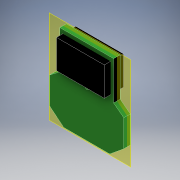
# Autodesk Inventor part: Probe
Saved by Autodesk Inventor 2020 (Build 240168000, 168)
## iProperties
Created: 2020-07-27
Part Number: Probe
Material: 일반
Document SubType Name: Modeling
Designer: Knowblesse
Density: 1 g/cm^3
Appearance: 기본값
Author: Knowblesse
Autodesk Inventor part; units mm, degrees
ref_plane "YZ Plane" through (0, 0, 0) normal (1, 0, 0) x (0, 1, 0)
ref_plane "XZ Plane" through (0, 0, 0) normal (0, 1, 0) x (-1, 0, 0)
ref_plane "XY Plane" through (0, 0, 0) normal (0, 0, 1) x (1, 0, 0)
sketch "스케치1" plane through (0, 0, 0) normal (0, 0, 1) x (1, 0, 0)
  line L0 (-3.5, -3) -> (3.5, -3)
  line L1 (3.5, -3) -> (3.5, 3)
  line L2 (3.5, 3) -> (-3.5, 3)
  line L3 (-3.5, 3) -> (-3.5, -3)
  line L4 (-3.5, -3) -> (3.5, 3) construction
  line L5 (3.5, -3) -> (-3.5, 3) construction
  line L6 (-4.825, -6.5) -> (4.825, -6.5)
  line L7 (4.825, -6.5) -> (4.825, -3)
  line L8 (4.825, -3) -> (-4.825, -3)
  line L9 (-4.825, -3) -> (-4.825, -6.5)
  line L10 (-4.825, -6.5) -> (4.825, -3) construction
  line L11 (4.825, -6.5) -> (-4.825, -3) construction
  line L12 (-4.825, -6.5) -> (-3, -8)
  line L13 (-3, -8) -> (3, -8)
  line L14 (3, -8) -> (4.825, -6.5)
  line L15 (4.825, -3) -> (3.5, -2)
  line L16 (-4.825, -3) -> (-3.5, -2)
  point P0 (0, 0)
  point P1 (0, -4.75)
  point P2 (0, -8)
  point P3 (0, -6.5)
  point P4 (0, 0)
  point P5 (0, -3)
  dimension "d0" = 7
  dimension "d1" = 6
  dimension "d2" = 9.65
  dimension "d3" = 3.5
  dimension "d4" = 1.5
  dimension "d5" = 6
  dimension "d7" = 1
  constraints: 34 end point, 9 midpoint, 4 parallel, 3 horizontal, 3 vertical alignment, 2 perpendicular, 2 point on line, 1 horizontal alignment
  measures "d0" distance of L2.end L1.end
  measures "d1" distance of L1.end L0.end
  measures "d2" distance of L8.end L7.end
  measures "d3" distance of L7.end L6.end
  measures "d4" distance between parallel lines of L6 L13
  measures "d5" distance of L12.end L13.end
  measures "d7" distance from line of L15.end L8
extrude "돌출1" add sketch "스케치1" along normal blind 0.85
ref_plane "작업 평면2" through (0, 0, 0.425) normal (0, 0, 1) x (1, 0, 0)
sketch "스케치4" plane through (0, 0, 0.425) normal (0, 0, 1) x (1, 0, 0)
  line L0 (3.11, 2.5) -> (-3.11, 2.5)
  line L1 (-3.11, 2.5) -> (-3.11, -1.26)
  line L2 (-3.11, -1.26) -> (3.11, -1.26)
  line L3 (3.11, -1.26) -> (3.11, 2.5)
  line L4 (3.5, 3) -> (-3.5, 3) projected
  point P0 (0, 0)
  point P1 (0, 2.5)
  dimension "d15" = 3.76
  dimension "d16" = 6.22
  dimension "d17" = 0.5
  constraints: 8 end point, 2 parallel, 1 horizontal, 1 midpoint, 1 perpendicular, 1 vertical alignment
  measures "d15" distance of L2.end L0.start
  measures "d16" distance of L0.start L0.end
  measures "d17" distance between parallel lines of L4 L0
extrude "돌출3" add sketch "스케치4" along normal mid plane 2.5 separate body
sketch "스케치5" plane through (0, 0, 0) normal (0, 0, -1) x (-1, 0, 0)
  line L0 (-3.5, 3) -> (3.5, 3) projected
  point P0 (-3.5, -2)
  point P1 (0, 0)
  point P2 (0, -2)
  point P3 (0, 3)
  constraints: 1 horizontal alignment, 1 midpoint, 1 vertical alignment
hole "구멍1" at (0, -2, 0) direction (0, 0, 1) diameter 0.5 end through all bodies 1
